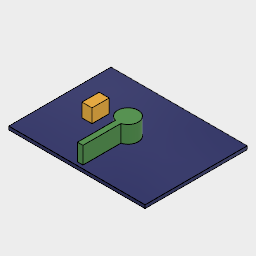
C04-W3-L2-03 v0 (Autodesk Fusion 360 design; units mm, degrees)
Autodesk Fusion 360 part; units mm, degrees
sketch "Sketch1" plane through (0, 0, 0) normal (0, 1, 0) x (1, 0, 0)
  line L0 (100, -75) -> (-100, -75)
  line L1 (-100, -75) -> (-100, 75)
  line L2 (-100, 75) -> (100, 75)
  line L3 (100, 75) -> (100, -75)
  line L4 (100, -75) -> (-100, 75) construction
  line L5 (-100, -75) -> (100, 75) construction
  circle A0 centre (0, 0) radius 10
  dimension "d1" = 200
  dimension "d2" = 150
  dimension "d3" = 20
  measures "d1" distance of L1.end L2.end
  measures "d2" distance of L0.start L2.end
  measures "d3" diameter of A0
extrude "Extrude1" add sketch "Sketch1" along normal blind 5 makes body 1
sketch "Sketch1 (2)" plane through (0, 5, 0) normal (0, 1, 0) x (-1, 0, 0) in component "Paddle"
  circle A0 centre (0, 0) radius 10
  line L0 (-100, -75) -> (100, -75)
  line L1 (100, -75) -> (100, 75)
  line L2 (100, 75) -> (-100, 75)
  line L3 (-100, 75) -> (-100, -75)
  circle A1 centre (0, 0) radius 10
  circle A2 centre (0, 0) radius 15
  line L4 (4, 14.4568) -> (4, 70)
  line L5 (4, 70) -> (-4, 70)
  line L6 (-4, 70) -> (-4, 14.4568)
  dimension "d6" = 20
  dimension "d7" = 30
  dimension "d8" = 4
  dimension "d9" = 8
  dimension "d10" = 70
  measures "d6" diameter of A1
  measures "d7" diameter of A2
  measures "d8" distance of A0.centre L6
  measures "d9" distance of L4 L6
  measures "d10" distance of A0.centre L5
extrude "Extrude1'" add sketch "Sketch1 (2)" against normal blind 5 separate body contours A0 A1 makes body 2 in component "Paddle"
extrude "Extrude2" add sketch "Sketch1 (2)" along normal blind 25 contours A0 A1 | A2 | A2 L4 L5 L6 bodies 2 in component "Paddle"
box "BoxPrimitive1" add length 25 width 14.6371 height 20 placed x (0, 0, 1) y (1, 0, 0) z (0, 1, 0) at (-56.5289, 5, -14.1597) separate body makes body 3 in component "Block"
component "Paddle" placed x (1, 0, 0) y (0, 1, 0) z (0, 0, 1) at (0, 0, 0)
component "Block" placed x (1, 0, 0) y (0, 1, 0) z (0, 0, 1) at (0, 0, 0)
named bodies: "Base Plate"
